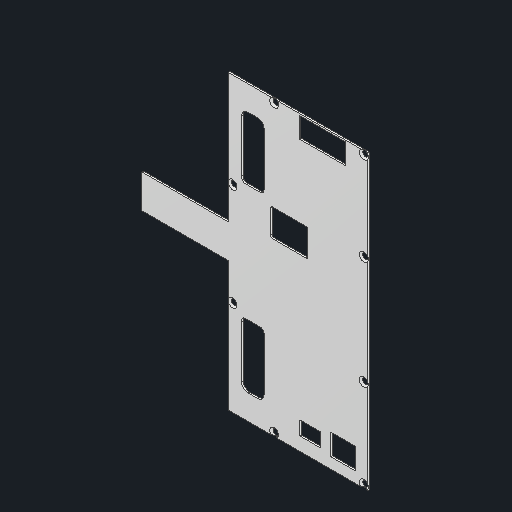
# Autodesk Inventor part: ceil
Saved by Autodesk Inventor 2023 (Build 270158000, 158)
## iProperties
Created: 2024-05-26
Part Number: ceil
Material: ABS Plastic
Document SubType Name: Modeling
Designer: szymo
Density: 1.06 g/cm^3
Appearance: Smooth - White
Mass: 14.8562 g
Surface Area: 292.494 cm^2
Volume: 14.0153 cm^3
Author: szymo
Autodesk Inventor part; units mm, degrees
ref_plane "YZ Plane" through (0, 0, 0) normal (1, 0, 0) x (0, 1, 0)
ref_plane "XZ Plane" through (0, 0, 0) normal (0, 1, 0) x (-1, 0, 0)
ref_plane "XY Plane" through (0, 0, 0) normal (0, 0, 1) x (1, 0, 0)
sketch "Sketch1" plane through (0, 0, 0) normal (0, 0, 1) x (1, 0, 0)
  arc A0 (81.0648, -49.5) -> (80.0648, -50.5) centre (81.0648, -50.5) ccw projected
  line L0 (80.0648, -52.5) -> (80.0648, -50.5) projected
  line L1 (35, -52.5) -> (80.0648, -52.5) projected
  line L2 (35, -52.5) -> (35, -50.5) projected
  arc A1 (30, -45.5) -> (35, -50.5) centre (35, -45.5) ccw projected
  line L3 (30, -45.5) -> (30, -37.5) projected
  line L4 (22.4833, -37.5) -> (30, -37.5) projected
  line L5 (22.4833, -47.5) -> (22.4833, -37.5) projected
  arc A2 (17.4833, -52.5) -> (22.4833, -47.5) centre (17.4833, -47.5) ccw projected
  line L6 (12.5167, -52.5) -> (17.4833, -52.5) projected
  arc A3 (7.5167, -47.5) -> (12.5167, -52.5) centre (12.5167, -47.5) ccw projected
  line L7 (7.5167, -47.5) -> (7.5167, -37.5) projected
  line L8 (0, -37.5) -> (7.5167, -37.5) projected
  line L9 (0, -53.5) -> (0, -37.5) projected
  line L10 (85.0648, -53.5) -> (0, -53.5) projected
  line L11 (85.0648, -53.5) -> (85.0648, -49.8187) projected
  arc A4 (85.0648, -49.8187) -> (84.3327, -49.5) centre (84.3327, -50.5) ccw projected
  line L12 (81.0648, -49.5) -> (84.3327, -49.5) projected
  circle A5 centre (82.5648, -51.5) radius 1.75 projected
  circle A6 centre (28, -51.5) radius 1.75 projected
  arc A7 (80.0648, 121.5) -> (81.0648, 120.5) centre (81.0648, 121.5) ccw projected
  line L13 (81.0648, 120.5) -> (84.3327, 120.5) projected
  arc A8 (84.3327, 120.5) -> (85.0648, 120.8187) centre (84.3327, 121.5) ccw projected
  line L14 (85.0648, 124.5) -> (85.0648, 120.8187) projected
  line L15 (85.0648, 124.5) -> (0, 124.5) projected
  line L16 (0, 124.5) -> (0, 108.5) projected
  line L17 (0, 108.5) -> (7.5167, 108.5) projected
  line L18 (7.5167, 118.5) -> (7.5167, 108.5) projected
  arc A9 (12.5167, 123.5) -> (7.5167, 118.5) centre (12.5167, 118.5) ccw projected
  line L19 (12.5167, 123.5) -> (17.4833, 123.5) projected
  arc A10 (22.4833, 118.5) -> (17.4833, 123.5) centre (17.4833, 118.5) ccw projected
  line L20 (22.4833, 118.5) -> (22.4833, 108.5) projected
  line L21 (22.4833, 108.5) -> (30, 108.5) projected
  line L22 (30, 116.5) -> (30, 108.5) projected
  arc A11 (35, 121.5) -> (30, 116.5) centre (35, 116.5) ccw projected
  line L23 (35, 123.5) -> (35, 121.5) projected
  line L24 (35, 123.5) -> (80.0648, 123.5) projected
  line L25 (80.0648, 123.5) -> (80.0648, 121.5) projected
  circle A12 centre (82.5648, 122.5) radius 1.75 projected
  circle A13 centre (28, 122.5) radius 1.75 projected
  line L26 (70.3148, 112) -> (70.3148, 123) projected
  line L27 (70.3148, 123) -> (44.3148, 123) projected
  line L28 (44.3148, 123) -> (44.3148, 112) projected
  line L29 (44.3148, 112) -> (70.3148, 112) projected
  line L30 (76.5648, -34.9) -> (63.5648, -34.9) projected
  line L31 (63.5648, -34.9) -> (63.5648, -45.9) projected
  line L32 (63.5648, -45.9) -> (76.5648, -45.9) projected
  line L33 (76.5648, -45.9) -> (76.5648, -34.9) projected
  line L34 (55.0648, -37.9) -> (44.5648, -37.9) projected
  line L35 (44.5648, -37.9) -> (44.5648, -44.4) projected
  line L36 (44.5648, -44.4) -> (55.0648, -44.4) projected
  line L37 (55.0648, -44.4) -> (55.0648, -37.9) projected
  circle A14 centre (2.676, 4.35) radius 1.75 projected
  circle A15 centre (82.5648, 2.5) radius 1.75 projected
  line L38 (0, 0) -> (85.0648, 0) projected
  line L39 (85.0648, 0) -> (85.0648, 5) projected
  line L40 (12.4976, 5) -> (85.0648, 5) projected
  arc A16 (5.352, 8.7) -> (12.4976, 5) centre (12.4976, 13.75) ccw projected
  line L41 (-52.5, 8.7) -> (5.352, 8.7) projected
  line L42 (-52.5, 5.7) -> (-52.5, 8.7) projected
  line L43 (-52.5, 5.7) -> (-49, 5.7) projected
  line L44 (-49, 5.7) -> (-3.5, 5.7) projected
  line L45 (-3.5, 5.7) -> (-2.1566, 5.7) projected
  arc A17 (-1.2313, 5.0793) -> (-2.1566, 5.7) centre (-2.1566, 4.7) ccw projected
  arc A18 (0, 0) -> (-1.2313, 5.0793) centre (-17.28, -1.5) ccw projected
  circle A19 centre (2.676, 66.65) radius 1.75 projected
  circle A20 centre (82.5648, 68.5) radius 1.75 projected
  line L46 (0, 71) -> (85.0648, 71) projected
  arc A21 (-1.2313, 65.9207) -> (0, 71) centre (-17.28, 72.5) ccw projected
  arc A22 (-2.1566, 65.3) -> (-1.2313, 65.9207) centre (-2.1566, 66.3) ccw projected
  line L47 (-3.5, 65.3) -> (-2.1566, 65.3) projected
  line L48 (-49, 65.3) -> (-3.5, 65.3) projected
  line L49 (-52.5, 65.3) -> (-49, 65.3) projected
  line L50 (-52.5, 65.3) -> (-52.5, 62.3) projected
  line L51 (-52.5, 62.3) -> (5.352, 62.3) projected
  arc A23 (12.4976, 66) -> (5.352, 62.3) centre (12.4976, 57.25) ccw projected
  line L52 (12.4976, 66) -> (85.0648, 66) projected
  line L53 (85.0648, 71) -> (85.0648, 66) projected
  arc A24 (-1, 24.3) -> (0, 25.3) centre (-1, 25.3) ccw projected
  line L54 (5.352, 25.3) -> (0, 25.3) projected
  line L55 (5.352, 28.3) -> (5.352, 25.3) projected
  line L56 (-52.5, 28.3) -> (5.352, 28.3) projected
  line L57 (-52.5, 28.3) -> (-52.5, 24.3) projected
  line L58 (-46.5, 24.3) -> (-52.5, 24.3) projected
  arc A25 (-46.5, 24.3) -> (-45.5, 25.3) centre (-46.5, 25.3) ccw projected
  line L59 (-7, 25.3) -> (-45.5, 25.3) projected
  arc A26 (-7, 25.3) -> (-6, 24.3) centre (-6, 25.3) ccw projected
  line L60 (-1, 24.3) -> (-6, 24.3) projected
  arc A27 (0, 45.7) -> (-1, 46.7) centre (-1, 45.7) ccw projected
  line L61 (-1, 46.7) -> (-6, 46.7) projected
  arc A28 (-6, 46.7) -> (-7, 45.7) centre (-6, 45.7) ccw projected
  line L62 (-7, 45.7) -> (-45.5, 45.7) projected
  arc A29 (-45.5, 45.7) -> (-46.5, 46.7) centre (-46.5, 45.7) ccw projected
  line L63 (-46.5, 46.7) -> (-52.5, 46.7) projected
  line L64 (-52.5, 42.7) -> (-52.5, 46.7) projected
  line L65 (-52.5, 42.7) -> (5.352, 42.7) projected
  line L66 (5.352, 42.7) -> (5.352, 45.7) projected
  line L67 (5.352, 45.7) -> (0, 45.7) projected
  line L68 (0, 124.5) -> (85.0648, 124.5)
  line L69 (85.0648, 124.5) -> (85.0648, -53.5)
  line L70 (85.0648, -53.5) -> (0, -53.5)
  line L71 (0, -53.5) -> (0, 124.5)
  line L72 (-52.5, 5.7) -> (0, 5.7)
  line L73 (0, 5.7) -> (0, 65.3)
  line L74 (0, 65.3) -> (-52.5, 65.3)
  line L75 (-52.5, 65.3) -> (-52.5, 5.7)
  line L76 (-52.5, 5.7) -> (0, 5.7)
  line L77 (0, 5.7) -> (0, 8.7)
  line L78 (0, 8.7) -> (-52.5, 8.7)
  line L79 (-52.5, 8.7) -> (-52.5, 5.7)
  line L80 (0, 45.7) -> (-52.5, 45.7)
  line L81 (-52.5, 45.7) -> (-52.5, 42.7)
  line L82 (-52.5, 42.7) -> (0, 42.7)
  line L83 (0, 42.7) -> (0, 45.7)
  line L84 (0, 65.3) -> (-52.5, 65.3)
  line L85 (-52.5, 65.3) -> (-52.5, 62.3)
  line L86 (-52.5, 62.3) -> (0, 62.3)
  line L87 (0, 62.3) -> (0, 65.3)
  line L88 (-52.5, 28.3) -> (0, 28.3)
  line L89 (0, 28.3) -> (0, 25.3)
  line L90 (0, 25.3) -> (-52.5, 25.3)
  line L91 (-52.5, 25.3) -> (-52.5, 28.3)
  line L92 (-52.5, 28.3) -> (0, 28.3)
  line L93 (0, 28.3) -> (0, 42.7)
  line L94 (0, 42.7) -> (-52.5, 42.7)
  line L95 (-52.5, 42.7) -> (-52.5, 28.3)
  line L96 (43.5648, -36.9) -> (56.0648, -36.9)
  line L97 (56.0648, -36.9) -> (56.0648, -45.4)
  line L98 (56.0648, -45.4) -> (43.5648, -45.4)
  line L99 (43.5648, -45.4) -> (43.5648, -36.9)
  line L100 (62.5648, -46.9) -> (62.5648, -33.9)
  line L101 (62.5648, -33.9) -> (77.5648, -33.9)
  line L102 (77.5648, -33.9) -> (77.5648, -46.9)
  line L103 (77.5648, -46.9) -> (62.5648, -46.9)
  line L104 (43.3148, 111) -> (43.3148, 124)
  line L105 (43.3148, 124) -> (71.3148, 124)
  line L106 (71.3148, 124) -> (71.3148, 111)
  line L107 (71.3148, 111) -> (43.3148, 111)
  line L108 (26.9124, 51.3) -> (47.4124, 51.3) projected
  ellipse E0 centre (26.9117, 51.3993) end of major axis (26.9821, 51.3289) minor radius 0.099 (26.8124, 51.4) -> (26.9124, 51.3) ccw projected
  line L109 (26.8124, 65.9) -> (26.8124, 51.4) projected
  ellipse E1 centre (26.9117, 65.9007) end of major axis (26.9821, 65.9711) minor radius 0.099 (26.9124, 66) -> (26.8124, 65.9) ccw projected
  ellipse E2 centre (47.4131, 51.3993) end of major axis (47.4835, 51.4697) minor radius 0.099 (47.4124, 51.3) -> (47.5124, 51.4) ccw projected
  line L110 (47.5124, 51.4) -> (47.5124, 65.9) projected
  ellipse E3 centre (47.4131, 65.9007) end of major axis (47.4835, 65.8303) minor radius 0.099 (47.5124, 65.9) -> (47.4124, 66) ccw projected
  line L111 (48.5124, 65.9001) -> (48.5124, 51.3999)
  line L112 (47.4125, 50.3) -> (26.9123, 50.3)
  line L113 (25.8124, 51.3999) -> (25.8124, 65.9001)
  line L114 (26.913, 67) -> (47.4125, 67)
  line L115 (20.8852, -3) -> (20.8852, -34.5) projected
  arc A30 (17.8852, -37.5) -> (20.8852, -34.5) centre (17.8852, -34.5) ccw projected
  line L116 (12.1148, -37.5) -> (17.8852, -37.5) projected
  arc A31 (9.1148, -34.5) -> (12.1148, -37.5) centre (12.1148, -34.5) ccw projected
  line L117 (9.1148, -3) -> (9.1148, -34.5) projected
  arc A32 (12.1148, 0) -> (9.1148, -3) centre (12.1148, -3) ccw projected
  line L118 (17.8852, 0) -> (12.1148, 0) projected
  arc A33 (20.8852, -3) -> (17.8852, 0) centre (17.8852, -3) ccw projected
  line L119 (9.1148, 74) -> (9.1148, 105.5) projected
  arc A34 (12.1148, 108.5) -> (9.1148, 105.5) centre (12.1148, 105.5) ccw projected
  line L120 (17.8852, 108.5) -> (12.1148, 108.5) projected
  arc A35 (20.8852, 105.5) -> (17.8852, 108.5) centre (17.8852, 105.5) ccw projected
  line L121 (20.8852, 74) -> (20.8852, 105.5) projected
  arc A36 (9.1148, 74) -> (12.1148, 71) centre (12.1148, 74) ccw projected
  arc A37 (17.8852, 71) -> (20.8852, 74) centre (17.8852, 74) ccw projected
  arc A38 (8.1148, -34.5) -> (12.1148, -38.5) centre (12.1148, -34.5) ccw
  line L122 (12.1148, -38.5) -> (17.8852, -38.5)
  arc A39 (17.8852, -38.5) -> (21.8852, -34.5) centre (17.8852, -34.5) ccw
  line L123 (21.8852, -34.5) -> (21.8852, -3)
  arc A40 (21.8852, -3) -> (17.8852, 1) centre (17.8852, -3) ccw
  line L124 (17.8852, 1) -> (12.1148, 1)
  arc A41 (12.1148, 1) -> (8.1148, -3) centre (12.1148, -3) ccw
  line L125 (8.1148, -3) -> (8.1148, -34.5)
  arc A42 (17.8852, 70) -> (21.8852, 74) centre (17.8852, 74) ccw
  line L126 (21.8852, 74) -> (21.8852, 105.5)
  arc A43 (21.8852, 105.5) -> (17.8852, 109.5) centre (17.8852, 105.5) ccw
  line L127 (17.8852, 109.5) -> (12.1148, 109.5)
  arc A44 (12.1148, 109.5) -> (8.1148, 105.5) centre (12.1148, 105.5) ccw
  line L128 (8.1148, 105.5) -> (8.1148, 74)
  arc A45 (8.1148, 74) -> (12.1148, 70) centre (12.1148, 74) ccw
  line L129 (12.1148, 70) -> (17.8852, 70)
  spline S0 degree 5 poles (47.4125, 67) (47.7581, 67.0001) (48.1038, 66.8645) (48.3769, 66.5914) (48.5125, 66.2457) (48.5124, 65.9001) knots 0 0 0 0 0 0 1 1 1 1 1 1
  spline S1 degree 5 poles (48.5124, 51.3999) (48.5125, 51.0543) (48.3769, 50.7086) (48.1038, 50.4355) (47.7581, 50.2999) (47.4125, 50.3) knots 0 0 0 0 0 0 1 1 1 1 1 1
  spline S2 degree 5 poles (26.9123, 50.3) (26.5667, 50.2999) (26.221, 50.4355) (25.9479, 50.7086) (25.8123, 51.0543) (25.8124, 51.3999) knots 0 0 0 0 0 0 1 1 1 1 1 1
  spline S3 degree 5 poles (25.8124, 65.9001) (25.8123, 66.2458) (25.948, 66.5917) (26.2213, 66.8648) (26.5672, 67.0003) (26.913, 67) knots 0 0 0 0 0 0 1 1 1 1 1 1
  point P0 (43.3148, 123.5)
  point P1 (71.3148, 123.5)
  point P2 (0, 25.3)
  point P3 (0, 45.7)
  point P4 (-7, 45.7)
  point P5 (48.5079, 66)
  point P6 (25.817, 66)
  point P7 (9.4691, 71)
  point P8 (20.5309, 71)
  point P9 (9.4691, 0)
  point P10 (20.5309, 0)
  dimension "d12" = 1
  dimension "d0" = 1
  dimension "d1" = 1
  dimension "d2" = 1
  dimension "d13" = 1
  dimension "d14" = 1
  constraints: 104 end point, 20 parallel, 16 point on circle, 9 horizontal, 8 centre point, 7 perpendicular, 3 point on line, 1 collinear, 38 other
  measures "d0" distance between parallel lines of L34 L96
  measures "d1" distance between parallel lines of L31 L100
  measures "d2" distance between parallel lines of L28 L104
  measures "d13" distance between parallel lines of L117 L125
  measures "d14" distance between parallel lines of L119 L128
extrude "Extrusion1" add sketch "Sketch1" along normal blind 1 contours L12 A4 L11 L10 L9 L8 L7 A3 L6 A2 L5 L4 L3 A1 L2 L1 L0 A0 | A0 L0 L1 L2 A1 L3 L4 L5 A2 L6 A3 L7 L8 L71 L38 A41 L125 A38 L122 A39 L123 A40 L69 A4 L12 | L38 A40 L124 A41 L71 L41 A16 L40 L39 | L38 A41 L124 A40 | L40 A16 L41 L71 L54 L55 L56 L65 L66 L67 L51 A23 L52 S3 L113 S2 L112 S1 L111 S0 L69 | L52 S0 L114 S3 A23 L51 L71 L46 A45 L129 A42 L53 | L46 A42 L126 A43 L127 A44 L128 A45 L71 L17 L18 A9 L19 A10 L20 L21 L22 A11 L23 L24 L104 L107 L106 L25 A7 L13 A8 L69 | A42 L129 A45 L46 | A8 L13 A7 L25 L24 L106 L105 L104 L23 A11 L22 L21 L20 A10 L19 A9 L18 L17 L16 L15 L14 | L71 L56 L55 L54 | L90 L59 L57 L56 L71 | L56 L75 L65 L71 | L71 L67 L66 L65 | L65 L64 L80 L62 L71 | L24 L104 L105 L106 | A5 | A6 | A12 | A13 | A14 | A15 | A19 | A20
sketch "Sketch2" plane through (0, 0, 1) normal (0, 0, 1) x (1, 0, 0)
  arc A0 (81.0648, -49.5) -> (80.0648, -50.5) centre (81.0648, -50.5) ccw projected
  line L0 (80.0648, -52.5) -> (80.0648, -50.5) projected
  line L1 (35, -52.5) -> (80.0648, -52.5) projected
  line L2 (35, -52.5) -> (35, -50.5) projected
  arc A1 (30, -45.5) -> (35, -50.5) centre (35, -45.5) ccw projected
  line L3 (30, -45.5) -> (30, -37.5) projected
  line L4 (22.4833, -37.5) -> (30, -37.5) projected
  line L5 (22.4833, -47.5) -> (22.4833, -37.5) projected
  arc A2 (17.4833, -52.5) -> (22.4833, -47.5) centre (17.4833, -47.5) ccw projected
  line L6 (12.5167, -52.5) -> (17.4833, -52.5) projected
  arc A3 (7.5167, -47.5) -> (12.5167, -52.5) centre (12.5167, -47.5) ccw projected
  line L7 (7.5167, -47.5) -> (7.5167, -37.5) projected
  line L8 (0, -37.5) -> (7.5167, -37.5) projected
  line L9 (0, -53.5) -> (0, -37.5) projected
  line L10 (85.0648, -53.5) -> (0, -53.5) projected
  line L11 (85.0648, -53.5) -> (85.0648, -49.8187) projected
  arc A4 (85.0648, -49.8187) -> (84.3327, -49.5) centre (84.3327, -50.5) ccw projected
  line L12 (81.0648, -49.5) -> (84.3327, -49.5) projected
  circle A5 centre (82.5648, -51.5) radius 1.75 projected
  circle A6 centre (28, -51.5) radius 1.75 projected
  circle A7 centre (2.676, 4.35) radius 1.75 projected
  circle A8 centre (82.5648, 2.5) radius 1.75 projected
  line L13 (0, 0) -> (85.0648, 0) projected
  line L14 (85.0648, 0) -> (85.0648, 5) projected
  line L15 (12.4976, 5) -> (85.0648, 5) projected
  arc A9 (5.352, 8.7) -> (12.4976, 5) centre (12.4976, 13.75) ccw projected
  line L16 (-52.5, 8.7) -> (5.352, 8.7) projected
  line L17 (-52.5, 5.7) -> (-52.5, 8.7) projected
  line L18 (-52.5, 5.7) -> (-49, 5.7) projected
  line L19 (-49, 5.7) -> (-3.5, 5.7) projected
  line L20 (-3.5, 5.7) -> (-2.1566, 5.7) projected
  arc A10 (-1.2313, 5.0793) -> (-2.1566, 5.7) centre (-2.1566, 4.7) ccw projected
  arc A11 (0, 0) -> (-1.2313, 5.0793) centre (-17.28, -1.5) ccw projected
  circle A12 centre (2.676, 66.65) radius 1.75 projected
  circle A13 centre (82.5648, 68.5) radius 1.75 projected
  line L21 (0, 71) -> (85.0648, 71) projected
  arc A14 (-1.2313, 65.9207) -> (0, 71) centre (-17.28, 72.5) ccw projected
  arc A15 (-2.1566, 65.3) -> (-1.2313, 65.9207) centre (-2.1566, 66.3) ccw projected
  line L22 (-3.5, 65.3) -> (-2.1566, 65.3) projected
  line L23 (-49, 65.3) -> (-3.5, 65.3) projected
  line L24 (-52.5, 65.3) -> (-49, 65.3) projected
  line L25 (-52.5, 65.3) -> (-52.5, 62.3) projected
  line L26 (-52.5, 62.3) -> (5.352, 62.3) projected
  arc A16 (12.4976, 66) -> (5.352, 62.3) centre (12.4976, 57.25) ccw projected
  line L27 (12.4976, 66) -> (85.0648, 66) projected
  line L28 (85.0648, 71) -> (85.0648, 66) projected
  arc A17 (80.0648, 121.5) -> (81.0648, 120.5) centre (81.0648, 121.5) ccw projected
  line L29 (81.0648, 120.5) -> (84.3327, 120.5) projected
  arc A18 (84.3327, 120.5) -> (85.0648, 120.8187) centre (84.3327, 121.5) ccw projected
  line L30 (85.0648, 124.5) -> (85.0648, 120.8187) projected
  line L31 (85.0648, 124.5) -> (0, 124.5) projected
  line L32 (0, 124.5) -> (0, 108.5) projected
  line L33 (0, 108.5) -> (7.5167, 108.5) projected
  line L34 (7.5167, 118.5) -> (7.5167, 108.5) projected
  arc A19 (12.5167, 123.5) -> (7.5167, 118.5) centre (12.5167, 118.5) ccw projected
  line L35 (12.5167, 123.5) -> (17.4833, 123.5) projected
  arc A20 (22.4833, 118.5) -> (17.4833, 123.5) centre (17.4833, 118.5) ccw projected
  line L36 (22.4833, 118.5) -> (22.4833, 108.5) projected
  line L37 (22.4833, 108.5) -> (30, 108.5) projected
  line L38 (30, 116.5) -> (30, 108.5) projected
  arc A21 (35, 121.5) -> (30, 116.5) centre (35, 116.5) ccw projected
  line L39 (35, 123.5) -> (35, 121.5) projected
  line L40 (35, 123.5) -> (80.0648, 123.5) projected
  line L41 (80.0648, 123.5) -> (80.0648, 121.5) projected
  circle A22 centre (82.5648, 122.5) radius 1.75 projected
  circle A23 centre (28, 122.5) radius 1.75 projected
  constraints: 8 coincident
hole "Hole1" at (82.5648, -51.5, 1) at (28, -51.5, 1) at (2.676, 4.35, 1) at (82.5648, 2.5, 1) at (82.5648, 68.5, 1) at (2.676, 66.65, 1) at (82.5648, 122.5, 1) at (28, 122.5, 1) direction (0, 0, -1) diameter 2.9 end through all countersink diameter 5.5 countersink angle 90 clearance for "Countersunk Flat Head Screw ISO 2009/7046" size "M2.5" standard "ISO"
fillet "Fillet1" radius 2 4 edges at (9.4691, 0, 0.5) (20.5309, 0, 0.5) (9.4691, 71, 0.5) (20.5309, 71, 0.5)
body "Solid1"
